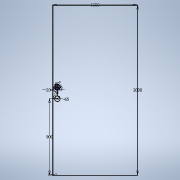
# Autodesk Inventor part: deadbolt arm
Saved by Autodesk Inventor 2022 (Build 260153000, 153)
## iProperties
Created: 2022-06-15
Part Number: deadbolt arm
Material: Generic
Document SubType Name: Modeling
Designer: alecw
Density: 1 g/cm^3
Appearance: Default
Author: alecw
Autodesk Inventor part; units mm, degrees
ref_plane "YZ Plane" through (0, 0, 0) normal (1, 0, 0) x (0, 1, 0)
ref_plane "XZ Plane" through (0, 0, 0) normal (0, 1, 0) x (-1, 0, 0)
ref_plane "XY Plane" through (0, 0, 0) normal (0, 0, 1) x (1, 0, 0)
sketch "Sketch1" plane through (0, 0, 0) normal (0, 0, 1) x (1, 0, 0)
  line L0 (0, 0) -> (1000, 0)
  line L1 (1000, 0) -> (1000, 2000)
  line L2 (1000, 2000) -> (0, 2000)
  line L3 (0, 2000) -> (0, 0)
  line L4 (0, 0) -> (4, 0)
  line L5 (0, 0) -> (4, 0) construction
  line L6 (4, 0) -> (4, 2000)
  line L7 (4, 0) -> (4, 900)
  line L8 (4, 900) -> (24, 900)
  line L9 (24, 900) -> (56.5, 900)
  circle A0 centre (56.5, 900) radius 32.5
  line L10 (56.5, 932.5) -> (56.5, 1002.5)
  line L11 (56.5, 1002.5) -> (56.5, 1036.1)
  circle A1 centre (56.5, 1036.1) radius 33.6
  line L12 (56.5, 1069.7) -> (56.5, 1037.7)
  line L13 (56.5, 1037.7) -> (56.5, 1064.7)
  line L14 (56.5, 1064.7) -> (56.5, 1028.7)
  line L15 (56.5, 1028.7) -> (56.5, 1010.7)
  line L16 (56.5, 1010.7) -> (58.505, 1010.7)
  line L17 (56.5, 1064.7) -> (58.505, 1064.7)
  line L18 (60.4989, 1062.8571) -> (63.008, 1031.0205)
  line L19 (60.478, 1012.372) -> (62.8086, 1026.3917)
  arc A2 (62.8086, 1026.3917) -> (63.008, 1031.0205) centre (43.9839, 1029.5211) ccw
  arc A3 (60.4989, 1062.8571) -> (58.505, 1064.7) centre (58.505, 1062.7) ccw
  arc A4 (58.505, 1010.7) -> (60.478, 1012.372) centre (58.505, 1012.7) ccw
  line L20 (63.0493, 1028.7) -> (56.5, 1028.7)
  line L21 (56.5, 1064.7) -> (54.495, 1064.7)
  line L22 (52.5011, 1062.8571) -> (49.992, 1031.0205)
  line L23 (52.522, 1012.372) -> (50.1914, 1026.3917)
  arc A5 (49.992, 1031.0205) -> (50.1914, 1026.3917) centre (69.0161, 1029.5211) ccw
  arc A6 (54.495, 1064.7) -> (52.5011, 1062.8571) centre (54.495, 1062.7) ccw
  arc A7 (52.522, 1012.372) -> (54.495, 1010.7) centre (54.495, 1012.7) ccw
  circle A8 centre (56.5, 1028.7) radius 5
  line L24 (56.5, 1010.7) -> (54.495, 1010.7)
  point P0 (60.2, 1010.7)
  point P1 (60.3536, 1064.7)
  point P2 (49.8, 1028.7)
  dimension "d11" = 65
  dimension "d0" = 1000
  dimension "d1" = 2000
  dimension "d2" = 4
  dimension "d8" = 900
  dimension "d9" = 20
  dimension "d10" = 32.5
  dimension "d12" = 70
  dimension "d13" = 33.6
  dimension "d24" = 32
  dimension "d25" = 27
  dimension "d26" = 36
  dimension "d27" = 18
  dimension "d28" = 3.7
  dimension "d31" = 2
  dimension "d32" = 6.5493
  dimension "d33" = 10
  constraints: 50 end point, 15 point on circle, 9 point on line, 9 symmetric about line, 8 centre point, 6 tangent, 5 horizontal, 5 vertical, 3 coincident, 3 perpendicular, 2 collinear, 2 equal length, 2 parallel, 1 equal radius, 1 vertical alignment, 5 other
  measures "d0" distance of L2.end L1.end
  measures "d1" distance of L1.end L0.end
  measures "d2" distance of L0.start L4.end
  measures "d8" distance of L5.end L7.end
  measures "d9" distance of L7.end L8.end
  measures "d10" distance of L8.end L9.end
  measures "d12" distance of L10.start L10.end
  measures "d13" distance of L10.end L11.end
  measures "d24" distance of L12.start L12.end
  measures "d25" distance of L12.end L13.end
  measures "d26" distance of L13.end L14.end
  measures "d27" distance of L14.end L15.end
  measures "d28" distance of L15.end point (60.2, 1010.7)
  measures "d31" radius of A3
  measures "d32" distance of L20.start L14.end
  measures "d33" diameter of A8
extrude "deadbolt axle" add sketch "Sketch1" along normal blind 2 contours A8 L11 | L11 L20 A8 | L11 A8 L20
extrude "deadbolt arm" add sketch "Sketch1" along normal blind 8 from surface at 2 contours L24 A7 L23 A5 L22 A6 L21 L12 L14 L11 A8 | L11 A8 L20 A2 L19 A4 L16 | A8 L11 | L11 L20 A8 | L17 A3 L18 A2 L20 A8 L11 L14 L12 | L11 A8 L20
body "Solid1"
